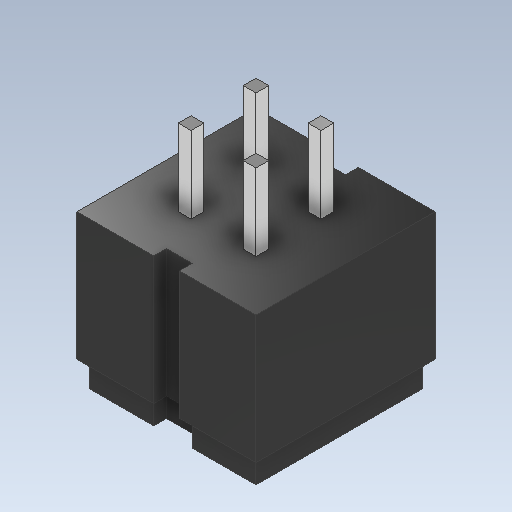
# Autodesk Inventor part: CNY70
Saved by Autodesk Inventor 2020 (Build 240168000, 168)
## iProperties
Created: 2020-03-26
Part Number: CNY70
Material: Generic
Document SubType Name: Modeling
Designer: ermoz
Density: 1 g/cm^3
Appearance: Default
Mass: 0.25875 g
Surface Area: 3.75418 cm^2
Volume: 0.25875 cm^3
Author: ermoz
Autodesk Inventor part; units mm, degrees
ref_plane "YZ Plane" through (0, 0, 0) normal (1, 0, 0) x (0, 1, 0)
ref_plane "XZ Plane" through (0, 0, 0) normal (0, 1, 0) x (-1, 0, 0)
ref_plane "XY Plane" through (0, 0, 0) normal (0, 0, 1) x (1, 0, 0)
sketch "Sketch1" plane through (0, 0, 0) normal (0, 1, 0) x (-1, 0, 0)
  line L0 (-3.5, -3.5) -> (3.5, -3.5)
  line L1 (3.5, -3.5) -> (3.5, 3.5)
  line L2 (3.5, 3.5) -> (-3.5, 3.5)
  line L3 (-3.5, 3.5) -> (-3.5, -3.5)
  line L4 (-3.5, -3.5) -> (3.5, 3.5) construction
  line L5 (3.5, -3.5) -> (-3.5, 3.5) construction
  point P0 (0, 0)
  dimension "d0" = 7
  dimension "d1" = 7
  constraints: 12 end point, 2 midpoint, 2 parallel, 1 horizontal, 1 perpendicular
  measures "d0" distance of L2.end L1.end
  measures "d1" distance of L1.end L0.end
extrude "Extrusion1" add sketch "Sketch1" along normal blind 6
sketch "Sketch2" plane through (0, 0, 0) normal (0, -1, 0) x (1, 0, 0)
  line L0 (-2.5, 2.5) -> (2.5, 2.5)
  line L1 (2.5, 2.5) -> (2.5, -2.5)
  line L2 (2.5, -2.5) -> (-2.5, -2.5)
  line L3 (-2.5, -2.5) -> (-2.5, 2.5)
  line L4 (-2.5, 2.5) -> (2.5, -2.5) construction
  line L5 (2.5, 2.5) -> (-2.5, -2.5) construction
  line L6 (-0.5, 4) -> (0.5, 4)
  line L7 (0.5, 4) -> (0.5, 3)
  line L8 (0.5, 3) -> (-0.5, 3)
  line L9 (-0.5, 3) -> (-0.5, 4)
  line L10 (-3.5, 3.5) -> (3.5, 3.5) projected
  line L11 (-0.5, 4) -> (0.5, 3) construction
  line L12 (0.5, 4) -> (-0.5, 3) construction
  line L13 (-0.5, -4) -> (0.5, -4)
  line L14 (0.5, -4) -> (0.5, -3)
  line L15 (0.5, -3) -> (-0.5, -3)
  line L16 (-0.5, -3) -> (-0.5, -4)
  line L17 (3.5, -3.5) -> (-3.5, -3.5) projected
  line L18 (-0.5, -4) -> (0.5, -3) construction
  line L19 (0.5, -4) -> (-0.5, -3) construction
  line L20 (-0.5, 3.5) -> (-3.5, 3.5)
  line L21 (-3.5, -3.5) -> (-3.5, 3.5) projected
  line L22 (-3.5, -3.5) -> (-3.5, 3.5)
  line L23 (-3.5, 3.5) -> (-3.5, -3.5)
  line L24 (-3.5, -3.5) -> (-0.5, -3.5)
  line L25 (0.5, -3.5) -> (3.5, -3.5)
  line L26 (3.5, -3.5) -> (3.5, 3.5)
  line L27 (3.5, 3.5) -> (0.5, 3.5)
  line L28 (3.5, 3.5) -> (3.5, -3.5) projected
  line L29 (3.5, 3.5) -> (3.5, -3.5)
  line L30 (3.25, -3.25) -> (-3.25, -3.25)
  line L31 (-3.25, -3.25) -> (-3.25, 3.25)
  line L32 (-3.25, 3.25) -> (3.25, 3.25)
  line L33 (3.25, 3.25) -> (3.25, -3.25)
  line L34 (3.25, -3.25) -> (-3.25, 3.25) construction
  line L35 (-3.25, -3.25) -> (3.25, 3.25) construction
  line L36 (-0.75, 3.75) -> (0.75, 3.75)
  line L37 (0.75, 3.75) -> (0.75, 2.75)
  line L38 (0.75, 2.75) -> (-0.75, 2.75)
  line L39 (-0.75, 2.75) -> (-0.75, 3.75)
  line L40 (-0.75, 3.75) -> (0.75, 2.75) construction
  line L41 (0.75, 3.75) -> (-0.75, 2.75) construction
  line L42 (-0.75, -3.75) -> (0.75, -3.75)
  line L43 (0.75, -3.75) -> (0.75, -2.75)
  line L44 (0.75, -2.75) -> (-0.75, -2.75)
  line L45 (-0.75, -2.75) -> (-0.75, -3.75)
  line L46 (-0.75, -3.75) -> (0.75, -2.75) construction
  line L47 (0.75, -3.75) -> (-0.75, -2.75) construction
  point P0 (0, 0)
  point P1 (0, 3.5)
  point P2 (0, -3.5)
  point P3 (0, 3.25)
  point P4 (0, -3.25)
  point P5 (-0.75, 3.25)
  point P6 (0.75, 3.25)
  point P7 (0.75, -3.25)
  point P8 (-0.75, -3.25)
  dimension "d10" = 6.5
  dimension "d11" = 6.5
  dimension "d12" = 1
  constraints: 88 end point, 20 midpoint, 12 parallel, 7 perpendicular, 7 point on line, 6 horizontal, 5 collinear
  measures "d10" distance of L31.end L32.end
  measures "d11" distance of L30.end L31.end
  measures "d12" distance of L36.end L37.end
extrude "Extrusion2" cut sketch "Sketch2" against normal blind 1 contours L0 L1 L2 L3 | L9 L32 L39 L10 | L10 L37 L32 L7 | L9 L8 L7 L32 L37 L38 L39 | L39 L32 L31 L30 L45 L17 L21 L10 | L10 L26 L17 L43 L30 L33 L32 L37 | L45 L30 L16 L17 | L17 L14 L30 L43 | L45 L44 L43 L30 L14 L15 L16
extrude "Extrusion3" cut sketch "Sketch2" against normal blind 10 contours L6 L7 L36 L9 | L36 L7 L10 L9 | L10 L7 L32 L9 | L32 L7 L8 L9 | L17 L14 L42 L16 | L16 L30 L14 L17 | L16 L15 L14 L30 | L42 L14 L13 L16
sketch "Sketch3" plane through (0, 6, 0) normal (0, 1, 0) x (1, 0, 0)
  line L0 (-1.4, -1.4) -> (1.4, -1.4)
  line L1 (1.4, -1.4) -> (1.4, 1.4)
  line L2 (1.4, 1.4) -> (-1.4, 1.4)
  line L3 (-1.4, 1.4) -> (-1.4, -1.4)
  line L4 (-1.4, -1.4) -> (1.4, 1.4) construction
  line L5 (1.4, -1.4) -> (-1.4, 1.4) construction
  line L6 (-1.65, 1.65) -> (-1.15, 1.65)
  line L7 (-1.15, 1.65) -> (-1.15, 1.15)
  line L8 (-1.15, 1.15) -> (-1.65, 1.15)
  line L9 (-1.65, 1.15) -> (-1.65, 1.65)
  line L10 (-1.65, 1.65) -> (-1.15, 1.15) construction
  line L11 (-1.15, 1.65) -> (-1.65, 1.15) construction
  line L12 (1.15, 1.65) -> (1.65, 1.65)
  line L13 (1.65, 1.65) -> (1.65, 1.15)
  line L14 (1.65, 1.15) -> (1.15, 1.15)
  line L15 (1.15, 1.15) -> (1.15, 1.65)
  line L16 (1.15, 1.65) -> (1.65, 1.15) construction
  line L17 (1.65, 1.65) -> (1.15, 1.15) construction
  line L18 (1.15, -1.15) -> (1.65, -1.15)
  line L19 (1.65, -1.15) -> (1.65, -1.65)
  line L20 (1.65, -1.65) -> (1.15, -1.65)
  line L21 (1.15, -1.65) -> (1.15, -1.15)
  line L22 (1.15, -1.15) -> (1.65, -1.65) construction
  line L23 (1.65, -1.15) -> (1.15, -1.65) construction
  line L24 (-1.65, -1.15) -> (-1.15, -1.15)
  line L25 (-1.15, -1.15) -> (-1.15, -1.65)
  line L26 (-1.15, -1.65) -> (-1.65, -1.65)
  line L27 (-1.65, -1.65) -> (-1.65, -1.15)
  line L28 (-1.65, -1.15) -> (-1.15, -1.65) construction
  line L29 (-1.15, -1.15) -> (-1.65, -1.65) construction
  point P0 (0, 0)
  dimension "d17" = 2.8
  dimension "d18" = 2.8
  dimension "d19" = 0.5
  dimension "d20" = 0.5
  dimension "d21" = 0.5
  dimension "d22" = 0.5
  dimension "d23" = 0.5
  dimension "d24" = 0.5
  dimension "d25" = 0.5
  dimension "d26" = 0.5
  constraints: 60 end point, 10 midpoint, 10 parallel, 5 horizontal, 5 perpendicular, 1 point on line
  measures "d17" distance of L2.end L1.end
  measures "d18" distance of L1.end L0.end
  measures "d19" distance of L7.end L8.end
  measures "d20" distance of L6.end L7.end
  measures "d21" distance of L13.end L14.end
  measures "d22" distance of L12.end L13.end
  measures "d23" distance of L19.end L20.end
  measures "d24" distance of L18.end L19.end
  measures "d25" distance of L25.end L26.end
  measures "d26" distance of L24.end L25.end
extrude "Extrusion4" add sketch "Sketch3" along normal blind 6 separate body contours L3 L24 L25 L0 | L0 L25 L26 L27 L24 L3 | L21 L18 L1 L0 | L0 L1 L18 L19 L20 L21 | L8 L9 L6 L7 L2 L3 | L3 L2 L7 L8 | L14 L15 L2 L1 | L1 L2 L15 L12 L13 L14
sketch "Sketch4" plane through (0, 12, 0) normal (0, 1, 0) x (1, 0, 0)
  line L0 (-1.27, 1.27) -> (1.27, 1.27)
  line L1 (1.27, 1.27) -> (1.27, -1.27)
  line L2 (1.27, -1.27) -> (-1.27, -1.27)
  line L3 (-1.27, -1.27) -> (-1.27, 1.27)
  line L4 (-1.27, 1.27) -> (1.27, -1.27) construction
  line L5 (1.27, 1.27) -> (-1.27, -1.27) construction
  line L6 (-1.52, -1.52) -> (-1.02, -1.52)
  line L7 (-1.02, -1.52) -> (-1.02, -1.02)
  line L8 (-1.02, -1.02) -> (-1.52, -1.02)
  line L9 (-1.52, -1.02) -> (-1.52, -1.52)
  line L10 (-1.52, -1.52) -> (-1.02, -1.02) construction
  line L11 (-1.02, -1.52) -> (-1.52, -1.02) construction
  line L12 (1.02, -1.52) -> (1.52, -1.52)
  line L13 (1.52, -1.52) -> (1.52, -1.02)
  line L14 (1.52, -1.02) -> (1.02, -1.02)
  line L15 (1.02, -1.02) -> (1.02, -1.52)
  line L16 (1.02, -1.52) -> (1.52, -1.02) construction
  line L17 (1.52, -1.52) -> (1.02, -1.02) construction
  line L18 (1.02, 1.52) -> (1.52, 1.52)
  line L19 (1.52, 1.52) -> (1.52, 1.02)
  line L20 (1.52, 1.02) -> (1.02, 1.02)
  line L21 (1.02, 1.02) -> (1.02, 1.52)
  line L22 (1.02, 1.52) -> (1.52, 1.02) construction
  line L23 (1.52, 1.52) -> (1.02, 1.02) construction
  line L24 (-1.52, 1.52) -> (-1.02, 1.52)
  line L25 (-1.02, 1.52) -> (-1.02, 1.02)
  line L26 (-1.02, 1.02) -> (-1.52, 1.02)
  line L27 (-1.52, 1.02) -> (-1.52, 1.52)
  line L28 (-1.52, 1.52) -> (-1.02, 1.02) construction
  line L29 (-1.02, 1.52) -> (-1.52, 1.02) construction
  line L30 (-1.945, 1.8515) -> (1.945, 1.8515)
  line L31 (1.945, 1.8515) -> (1.945, -1.8515)
  line L32 (1.945, -1.8515) -> (-1.945, -1.8515)
  line L33 (-1.945, -1.8515) -> (-1.945, 1.8515)
  line L34 (-1.945, 1.8515) -> (1.945, -1.8515) construction
  line L35 (1.945, 1.8515) -> (-1.945, -1.8515) construction
  point P0 (0, 0)
  dimension "d29" = 2.54
  dimension "d30" = 2.54
  dimension "d31" = 0.5
  dimension "d32" = 0.5
  dimension "d33" = 0.5
  dimension "d34" = 0.5
  dimension "d35" = 0.5
  dimension "d36" = 0.5
  dimension "d37" = 0.5
  dimension "d38" = 0.5
  constraints: 72 end point, 12 midpoint, 12 parallel, 6 horizontal, 6 perpendicular
  measures "d29" distance of L1.end L2.end
  measures "d30" distance of L0.end L1.end
  measures "d31" distance of L8.end L7.end
  measures "d32" distance of L7.end L6.end
  measures "d33" distance of L14.end L13.end
  measures "d34" distance of L13.end L12.end
  measures "d35" distance of L19.end L20.end
  measures "d36" distance of L18.end L19.end
  measures "d37" distance of L25.end L26.end
  measures "d38" distance of L24.end L25.end
extrude "Extrusion5" cut sketch "Sketch4" against normal blind 6 contours L3 L26 L27 L24 L25 L0 | L0 L25 L26 L3 | L0 L21 L20 L1 L14 L15 L2 L7 L8 L3 L26 L25 | L21 L18 L19 L20 L1 L0 | L0 L1 L20 L21 | L8 L7 L2 L3 | L3 L2 L7 L6 L9 L8 | L14 L13 L12 L15 L2 L1 | L1 L2 L15 L14 | L30 L31 L32 L33 bodies 2
extrude "Extrusion6" add sketch "Sketch4" against normal blind 6 separate body contours L3 L26 L27 L24 L25 L0 | L0 L25 L26 L3 | L21 L18 L19 L20 L1 L0 | L0 L1 L20 L21 | L8 L7 L2 L3 | L3 L2 L7 L6 L9 L8 | L14 L13 L12 L15 L2 L1 | L1 L2 L15 L14
sketch "Sketch5" plane through (0, 1, 0) normal (0, -1, 0) x (1, 0, 0)
  line L0 (0, 0) -> (-1.4, 0)
  line L1 (0, 0) -> (1.4, 0)
  circle A0 centre (-1.4, 0) radius 0.9
  circle A1 centre (1.4, 0) radius 0.9
  dimension "d43" = 1.4
  dimension "d44" = 1.4
  dimension "d45" = 1.8
  dimension "d46" = 1.8
  constraints: 4 end point, 2 centre point, 2 coincident, 2 horizontal
  measures "d43" distance of L0.start L0.end
  measures "d44" distance of L0.start L1.end
  measures "d45" diameter of A0
  measures "d46" diameter of A1
extrude "Extrusion7" cut sketch "Sketch5" against normal blind 2 bodies 1
extrude "Extrusion8" add sketch "Sketch5" against normal blind 2 separate body contours A1
extrude "Extrusion9" add sketch "Sketch5" against normal blind 2 separate body contours A0
sketch "Sketch6" plane through (0, 12, 0) normal (0, 1, 0) x (1, 0, 0)
  line L0 (-5.946, 4.9955) -> (6.4952, 4.9955)
  line L1 (6.4952, 4.9955) -> (6.4952, -3.9816)
  line L2 (6.4952, -3.9816) -> (-5.946, -3.9816)
  line L3 (-5.946, -3.9816) -> (-5.946, 4.9955)
  point P0 (0, 0)
  constraints: 8 end point, 2 parallel, 1 horizontal, 1 perpendicular
extrude "Extrusion10" cut sketch "Sketch6" against normal blind 3 bodies 3
body "Solid1"
body "Solid2"
body "Solid3"
body "Solid4"
body "Solid5"
